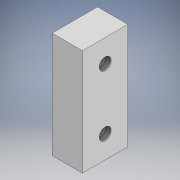
# Autodesk Inventor part: Threaded Block
Saved by Autodesk Inventor 2020 (Build 240168000, 168)
## iProperties
Created: 2019-09-11
Part Number: Threaded Block
Material: Generic
Document SubType Name: Modeling
Designer: Matt
Density: 1 g/cm^3
Appearance: Default
Author: Matt
Autodesk Inventor part; units mm, degrees
ref_plane "YZ Plane" through (0, 0, 0) normal (1, 0, 0) x (0, 1, 0)
ref_plane "XZ Plane" through (0, 0, 0) normal (0, 1, 0) x (-1, 0, 0)
ref_plane "XY Plane" through (0, 0, 0) normal (0, 0, 1) x (1, 0, 0)
sketch "Sketch1" plane through (0, 0, 0) normal (1, 0, 0) x (0, 1, 0)
  line L0 (-22.225, 9.525) -> (22.225, 9.525)
  line L1 (22.225, 9.525) -> (22.225, -9.525)
  line L2 (22.225, -9.525) -> (-22.225, -9.525)
  line L3 (-22.225, -9.525) -> (-22.225, 9.525)
  line L4 (-22.225, 9.525) -> (22.225, -9.525) construction
  line L5 (22.225, 9.525) -> (-22.225, -9.525) construction
  point P0 (0, 0)
  dimension "d0" = 44.45
  dimension "d1" = 19.05
  constraints: 12 end point, 2 midpoint, 2 parallel, 1 horizontal, 1 perpendicular
  measures "d0" distance of L1.end L2.end
  measures "d1" distance of L0.end L1.end
extrude "Extrusion1" add sketch "Sketch1" along normal blind 12.7
sketch "Sketch2" plane through (12.7, 0, 0) normal (1, 0, 0) x (0, 0, -1)
  circle A0 centre (0, 12.7) radius 3.3782
  circle A1 centre (0, -12.7) radius 3.3782
  line L0 (-660.4, 0) -> (-660.4, 41.275)
  line L1 (-9.525, 22.225) -> (-9.525, -22.225) projected
  line L2 (-12.7, 22.225) -> (-12.7, -22.225)
  point P0 (0, 0)
  dimension "d4" = 3.175
  dimension "d5" = 12.7
  constraints: 4 end point, 2 centre point, 1 parallel
  measures "d4" distance between parallel lines of L1 L2
  measures "d5" distance of point (0, 0) point (0, 12.7)
hole "Hole1" at (12.7, 12.7, 0) at (12.7, -12.7, 0) direction (-1, 0, 0) diameter 4.9784 end through all thread size "1/4-20 UNC" class "2B" standard "ANSI Unified Screw Threads"
body "Solid1"
